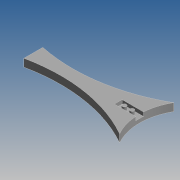
# Autodesk Inventor part: 3
Saved by Autodesk Inventor 2017 (Build 210142000, 142)
## iProperties
Created: 2018-10-12
Part Number: 3
Material: Générique
Document SubType Name: Modeling
Designer: Gilles Mottiez
Density: 1 g/cm^3
Appearance: Par défaut
Description: Balancier de dos
Author: Gilles Mottiez
Autodesk Inventor part; units mm, degrees
ref_plane "YZ Plane" through (0, 0, 0) normal (1, 0, 0) x (0, 1, 0)
ref_plane "XZ Plane" through (0, 0, 0) normal (0, 1, 0) x (-1, 0, 0)
ref_plane "XY Plane" through (0, 0, 0) normal (0, 0, 1) x (1, 0, 0)
sketch "Sketch1" plane through (0, 0, 0) normal (0, 0, 1) x (1, 0, 0)
  circle A0 centre (0, 0) radius 12.5 construction
  line L0 (0, 0) -> (140, 0) construction
  line L1 (140, 0) -> (210.5, 0) construction
  circle A1 centre (210.5, 0) radius 70.5 construction
  arc A2 (2.574, 12.2321) -> (149.3016, 35) centre (45.8166, 217.7317) ccw construction
  arc A3 (149.3016, -35) -> (2.574, -12.2321) centre (45.8166, -217.7317) ccw construction
  line L2 (2.574, 12.2321) -> (2.574, -12.2321)
  arc A4 (2.574, 12.2321) -> (149.3016, 35) centre (45.8166, 217.7317) ccw
  arc A5 (149.3016, -35) -> (2.574, -12.2321) centre (45.8166, -217.7317) ccw
  arc A6 (149.3016, 35) -> (149.3016, -35) centre (210.5, 0) ccw
  dimension "d0" = 25
  dimension "d1" = 140
  dimension "d2" = 70.5
  dimension "d3" = 210
  dimension "d4" = 35
  constraints: 15 point on circle, 7 centre point, 6 end point, 3 concentric, 2 coincident, 2 horizontal, 2 vertical alignment, 1 tangent, 1 vertical, 1 other
  measures "d0" diameter of A0
  measures "d1" distance of L0.start L0.end
  measures "d2" distance of L0.end L1.end
  measures "d3" radius of A2
  measures "d4" distance from line of A1.end L1
extrude "Extrusion1" add sketch "Sketch1" against normal blind 10
sketch "Esquisse2" plane through (0, 0, 0) normal (0, 0, 1) x (1, 0, 0)
  line L0 (2.574, 12.2321) -> (2.574, -12.2321) construction
  arc A0 (149.3016, -35) -> (2.574, -12.2321) centre (45.8166, -217.7317) ccw construction
  arc A1 (149.3016, 35) -> (149.3016, -35) centre (210.5, 0) ccw construction
  arc A2 (2.574, 12.2321) -> (149.3016, 35) centre (45.8166, 217.7317) ccw construction
  line L1 (210.5, 0) -> (0, 0) construction
  line L2 (140.5, 5) -> (112.5, 5) construction
  line L3 (112.5, 5) -> (112.5, -5) construction
  line L4 (112.5, -5) -> (140.5, -5) construction
  line L5 (140.5, -5) -> (140.5, 5) construction
  circle A3 centre (130.5, 0) radius 2.5
  circle A4 centre (120.5, 0) radius 2.5
  line L6 (140.5, 5) -> (112.5, 5)
  line L7 (112.5, 5) -> (112.5, -5)
  line L8 (112.5, -5) -> (140.5, -5)
  line L9 (140.5, -5) -> (140.5, 5)
  dimension "d7" = 28
  dimension "d8" = 10
  dimension "d9" = 70
  dimension "d10" = 5
  dimension "d11" = 5
  dimension "d12" = 10
  dimension "d13" = 80
  constraints: 18 end point, 5 equal length, 2 centre point, 2 horizontal, 2 perpendicular, 2 point on line, 1 other
  measures "d7" distance of L4.end L3.end
  measures "d8" distance of L3.end L2.end
  measures "d9" distance from line of L1.start L5
  measures "d10" diameter of A3
  measures "d11" diameter of A4
  measures "d12" distance of A4.centre A3.centre
  measures "d13" distance of L1.start A3.centre
extrude "Extrusion2" cut sketch "Esquisse2" against normal blind 5
